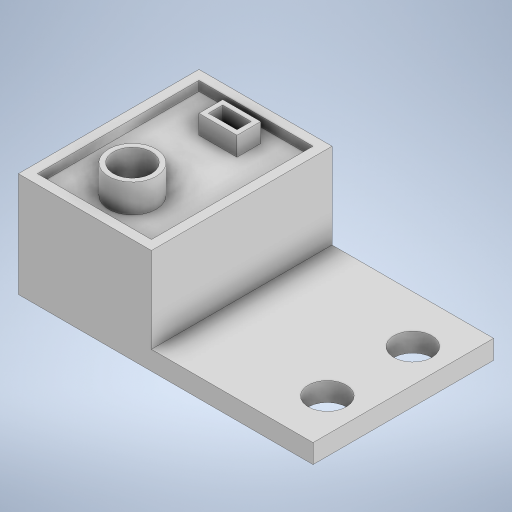
# Autodesk Inventor part: Deck_neu
Saved by Autodesk Inventor 2023 (Build 270158000, 158)
## iProperties
Created: 2023-03-30
Part Number: Deck_neu
Material: Generisch
Document SubType Name: Modeling
Designer: prigge
Density: 1 g/cm^3
Appearance: Vorgabe
Author: prigge
Autodesk Inventor part; units mm, degrees
ref_plane "YZ Plane" through (0, 0, 0) normal (1, 0, 0) x (0, 1, 0)
ref_plane "XZ Plane" through (0, 0, 0) normal (0, 1, 0) x (-1, 0, 0)
ref_plane "XY Plane" through (0, 0, 0) normal (0, 0, 1) x (1, 0, 0)
sketch "Skizze1" plane through (0, 0, 0) normal (0, 0, 1) x (1, 0, 0)
  line L0 (0, 0) -> (0, 2)
  line L1 (0, 2) -> (-17, 2)
  line L2 (-17, 2) -> (-17, 10)
  line L3 (-17, 10) -> (-31, 10)
  line L4 (-31, 10) -> (-31, 0)
  line L5 (-31, 0) -> (0, 0)
  dimension "d0" = 17
  dimension "d1" = 2
  dimension "d2" = 14
  dimension "d3" = 10
  constraints: 12 end point, 5 perpendicular, 1 vertical
  measures "d0" distance between parallel lines of L0 L2
  measures "d1" distance of L0.start L0.end
  measures "d2" distance of L2.end L3.end
  measures "d3" distance of L3.end L4.end
extrude "Extrusion1" add sketch "Skizze1" along normal mid plane 19
sketch "Skizze2" plane through (-31, 10, 9.5) normal (0, 1, 0) x (1, 0, 0)
  circle A0 centre (7, 5) radius 2.5
  line L0 (14, 0) -> (0, 0) projected
  point P0 (31, 9.5)
  point P1 (7, 0)
  dimension "d6" = 5
  dimension "d7" = 5
  constraints: 1 centre point, 1 midpoint, 1 vertical alignment
  measures "d6" diameter of A0
  measures "d7" distance from line of L0 A0.centre
extrude "Extrusion2" add sketch "Skizze2" along normal blind 3
sketch "Skizze3" plane through (-24, 13, 4.5) normal (0, 1, 0) x (1, 0, 0)
  circle A0 centre (0, 0) radius 2
  point P0 (24, 4.5)
  dimension "d10" = 4
  constraints: 1 centre point
  measures "d10" diameter of A0
extrude "Extrusion3" cut sketch "Skizze3" against normal through all
sketch "Skizze4" plane through (-31, 10, 9.5) normal (0, 1, 0) x (1, 0, 0)
  line L0 (5.5, 14.5) -> (8.5, 14.5)
  line L1 (8.5, 14.5) -> (8.5, 16)
  line L2 (8.5, 16) -> (5.5, 16)
  line L3 (5.5, 16) -> (5.5, 14.5)
  line L4 (0, 19) -> (14, 19) projected
  point P0 (31, 9.5)
  point P1 (7, 16)
  point P2 (7, 19)
  dimension "d13" = 1.5
  dimension "d14" = 3
  dimension "d15" = 3
  constraints: 8 end point, 2 midpoint, 2 parallel, 1 horizontal, 1 perpendicular, 1 vertical alignment
  measures "d13" distance of L2.end L0.start
  measures "d14" distance of L1.end L2.end
  measures "d15" distance between parallel lines of L4 L2
extrude "Extrusion4" cut sketch "Skizze4" against normal through all
sketch "Skizze5" plane through (-31, 10, 9.5) normal (0, 1, 0) x (1, 0, 0)
  line L0 (5.5, 16) -> (8.5, 16) projected
  line L1 (5, 14) -> (9, 14)
  line L2 (9, 14) -> (9, 16.5)
  line L3 (9, 16.5) -> (5, 16.5)
  line L4 (5, 16.5) -> (5, 14)
  line L5 (5.5, 14.5) -> (5.5, 16) projected
  line L6 (8.5, 16) -> (8.5, 14.5) projected
  line L7 (8.5, 14.5) -> (5.5, 14.5) projected
  point P0 (31, 9.5)
  point P1 (5, 15.25)
  point P2 (5.5, 15.25)
  point P3 (7, 14)
  point P4 (7, 16)
  dimension "d18" = 0.5
  dimension "d19" = 0.5
  constraints: 8 end point, 4 midpoint, 2 parallel, 1 horizontal, 1 horizontal alignment, 1 perpendicular, 1 vertical alignment
  measures "d18" distance between parallel lines of L3 L0
  measures "d19" distance between parallel lines of L4 L5
extrude "Extrusion5" add sketch "Skizze5" along normal blind 2
sketch "Skizze6" plane through (-31, 10, 9.5) normal (0, 1, 0) x (1, 0, 0)
  line L0 (0, 19) -> (0, 0) projected
  line L1 (0, 19) -> (14, 19) projected
  line L2 (14, 19) -> (14, 0) projected
  line L3 (14, 0) -> (0, 0) projected
  line L4 (1, 1) -> (13, 1)
  line L5 (13, 1) -> (13, 18)
  line L6 (13, 18) -> (1, 18)
  line L7 (1, 18) -> (1, 1)
  point P0 (31, 9.5)
  point P1 (1, 9.5)
  point P2 (0, 9.5)
  point P3 (7, 18)
  point P4 (7, 19)
  dimension "d22" = 1
  dimension "d23" = 1
  constraints: 8 end point, 4 midpoint, 2 parallel, 1 horizontal, 1 horizontal alignment, 1 perpendicular, 1 vertical alignment
  measures "d22" distance between parallel lines of L0 L7
  measures "d23" distance between parallel lines of L1 L6
extrude "Extrusion6" add sketch "Skizze6" along normal blind 1
sketch "Skizze7" plane through (-17, 2, 9.5) normal (0, 1, 0) x (1, 0, 0)
  line L0 (17, 19) -> (17, 0) projected
  line L1 (17, 19) -> (17, 14)
  line L2 (17, 14) -> (13.5, 14)
  line L3 (17, 0) -> (17, 5)
  line L4 (17, 5) -> (13.5, 5)
  point P0 (17, 9.5)
  dimension "d26" = 5
  dimension "d27" = 3.5
  dimension "d28" = 5
  dimension "d29" = 3.5
  constraints: 8 end point, 2 coincident, 2 perpendicular, 2 point on line
  measures "d26" distance of L0.start L1.end
  measures "d27" distance of L1.end L2.end
  measures "d28" distance of L0.end L3.end
  measures "d29" distance of L3.end L4.end
hole "Bohrung1" at (-3.5, 2, 4.5) at (-3.5, 2, -4.5) direction (0, -1, 0) diameter 4 depth 50 tip angle 118
